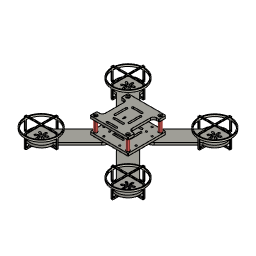
drone v11 (Autodesk Fusion 360 design; units mm, degrees)
Autodesk Fusion 360 part; units mm, degrees
(part 1 of 2)
sketch "Sketch1" plane through (0, 0, 0) normal (0, 0, 1) x (1, 0, 0)
  line L0 (0, 0) -> (74.2462, 0)
  line L1 (74.2462, 0) -> (74.2462, 74.2462)
  line L2 (74.2462, 74.2462) -> (0, 74.2462)
  line L3 (0, 74.2462) -> (0, 0)
  circle A0 centre (74.2462, 74.2462) radius 1
  circle A1 centre (0, 74.2462) radius 1
  circle A2 centre (0, 0) radius 1
  circle A3 centre (74.2462, 0) radius 1
  circle A4 centre (0, 74.2462) radius 10
  circle A5 centre (74.2462, 74.2462) radius 10
  circle A6 centre (74.2462, 0) radius 10
  circle A7 centre (0, 0) radius 10
  line L4 (59.6231, 14.6231) -> (14.6231, 14.6231)
  line L5 (14.6231, 14.6231) -> (14.6231, 59.6231)
  line L6 (14.6231, 59.6231) -> (59.6231, 59.6231)
  line L7 (59.6231, 59.6231) -> (59.6231, 14.6231)
  line L8 (59.6231, 14.6231) -> (14.6231, 59.6231) construction
  line L9 (14.6231, 14.6231) -> (59.6231, 59.6231) construction
  line L10 (0, 64.2462) -> (14.8037, 49.4426)
  line L11 (0, 64.2462) -> (20.9355, 64.2462) construction
  line L12 (10, 74.2462) -> (24.628, 59.6182)
  line L13 (10, 74.2462) -> (30.6871, 74.2462) construction
  line L14 (10, 0) -> (25.5198, 15.5198)
  line L15 (10, 0) -> (31.9483, 0) construction
  line L16 (0, 10) -> (14.6231, 24.6231)
  line L17 (0, 10) -> (20.6802, 10) construction
  line L18 (64.2462, 0) -> (49.6231, 14.6231)
  line L19 (74.2462, 10) -> (59.6231, 24.6231)
  line L20 (74.2462, 10) -> (94.9264, 10) construction
  line L21 (74.2462, 64.2462) -> (59.6231, 49.6231)
  line L22 (74.2462, 64.2462) -> (94.9264, 64.2462) construction
  line L23 (64.2462, 74.2462) -> (49.6231, 59.6231)
  line L24 (64.2462, 74.2462) -> (84.9264, 74.2462) construction
  point P0 (37.1231, 37.1231)
  dimension "d1" = 105
  dimension "d2" = 2
  dimension "d3" = 2
  dimension "d4" = 2
  dimension "d5" = 2
  dimension "d6" = 20
  dimension "d7" = 20
  dimension "d8" = 20
  dimension "d9" = 20
  dimension "d10" = 45
  dimension "d11" = 45
  dimension "d12" = 45
  constraint horizontal L0
  constraint vertical L1
  constraint horizontal L2
  constraint vertical L3
  constraint coincident L0.start L3.end
  constraint coincident L1.end L2.start
  constraint coincident L2.end L3.start
  constraint coincident L0.end L1.start
  constraint concentric A1 A4
  constraint concentric A0 A5
  constraint concentric A3 A6
  constraint concentric A2 A7
  constraint horizontal L4
  constraint perpendicular L4 L5
  constraint parallel L4 L6
  constraint parallel L5 L7
  constraint coincident L8 P0
  constraint coincident L9 P0
  constraint horizontal L11
  constraint coincident A4 L10.start
  constraint coincident L3 L10.start
  constraint horizontal L13
  constraint coincident A4 L12.start
  constraint coincident L2 L12.start
  constraint horizontal L15
  constraint coincident A7 L14.start
  constraint coincident L0 L14.start
  constraint horizontal L17
  constraint coincident A7 L16.start
  constraint coincident L3 L16.start
  constraint coincident L5 L16.end
  constraint coincident A6 L18.start
  constraint coincident L0 L18.start
  constraint coincident L4 L18.end
  constraint horizontal L20
  constraint coincident A6 L19.start
  constraint coincident L1 L19.start
  constraint coincident L7 L19.end
  constraint horizontal L22
  constraint coincident A5 L21.start
  constraint coincident L1 L21.start
  constraint coincident L7 L21.end
  constraint horizontal L24
  constraint coincident A5 L23.start
  constraint coincident L2 L23.start
  constraint coincident L6 L23.end
  measures "d1" distance of L0.start L1.end
  measures "d2" diameter of A0
  measures "d3" diameter of A1
  measures "d4" diameter of A2
  measures "d5" diameter of A3
  measures "d6" diameter of A4
  measures "d7" diameter of A5
  measures "d8" diameter of A6
  measures "d9" diameter of A7
  measures "d10" distance of L5.end L6.end
  measures "d11" distance of L4.end L5.end
  measures "d12" angle of L10 L11
extrude "Extrude1" add sketch "Sketch1" along normal blind 2 contours L0 L3 A2 A7 | L0 L3 A2 A7 | A7 L4 L5 L14 L16 | L0 L1 A3 A6 | A6 L4 L7 L18 L19 | L0 L1 A3 A6 | L4 L5 L6 L7 | L2 L3 A1 A4 | L2 L3 A1 A4 | A4 L5 L6 L10 L12 | L1 L2 A0 A5 | A5 L6 L7 L21 L23 | L1 L2 A0 A5 makes body 1
sketch "Sketch2" plane through (0, 0, 2) normal (0, 0, 1) x (-1, 0, 0)
  circle A0 centre (-74.2462, 0) radius 1
  circle A1 centre (0, -74.2462) radius 1
  circle A2 centre (0, 0) radius 1
  circle A3 centre (-74.2462, -74.2462) radius 1
  arc A4 (-74.2462, -64.2462) -> (-64.2462, -74.2462) centre (-74.2462, -74.2462) ccw
  line L0 (-64.2462, -74.2462) -> (-49.6231, -59.6231)
  line L1 (-49.6231, -59.6231) -> (-24.6231, -59.6231)
  line L2 (-24.6231, -59.6231) -> (-10, -74.2462)
  arc A5 (-10, -74.2462) -> (0, -64.2462) centre (0, -74.2462) ccw
  line L3 (0, -64.2462) -> (-14.6231, -49.6231)
  line L4 (-14.6231, -49.6231) -> (-14.6231, -24.6231)
  line L5 (-14.6231, -24.6231) -> (0, -10)
  arc A6 (0, -10) -> (-10, 0) centre (0, 0) ccw
  line L6 (-10, 0) -> (-24.6231, -14.6231)
  line L7 (-24.6231, -14.6231) -> (-49.6231, -14.6231)
  line L8 (-49.6231, -14.6231) -> (-64.2462, 0)
  arc A7 (-64.2462, 0) -> (-74.2462, -10) centre (-74.2462, 0) ccw
  line L9 (-74.2462, -10) -> (-59.6231, -24.6231)
  line L10 (-59.6231, -24.6231) -> (-59.6231, -49.6231)
  line L11 (-59.6231, -49.6231) -> (-74.2462, -64.2462)
  line L12 (0.7, -78.2462) -> (0.7, -76.5)
  arc A8 (0.7, -76.5) -> (-0.7, -76.5) centre (0, -76.5) ccw
  line L13 (-0.7, -76.5) -> (-0.7, -78.2462)
  arc A9 (-0.7, -78.2462) -> (0.7, -78.2462) centre (0, -78.2462) ccw
  line L14 (0, -78.2462) -> (0, -76.5) construction
  line L15 (3.8141, -75.64) -> (2.3018, -74.7669)
  arc A10 (3.1141, -76.8524) -> (3.8141, -75.64) centre (3.4641, -76.2462) ccw
  line L16 (1.6018, -75.9793) -> (3.1141, -76.8524)
  arc A11 (2.3018, -74.7669) -> (1.6018, -75.9793) centre (1.9518, -75.3731) ccw
  line L17 (3.1141, -71.64) -> (1.6018, -72.5131)
  arc A12 (3.8141, -72.8524) -> (3.1141, -71.64) centre (3.4641, -72.2462) ccw
  line L18 (2.3018, -73.7255) -> (3.8141, -72.8524)
  arc A13 (1.6018, -72.5131) -> (2.3018, -73.7255) centre (1.9518, -73.1193) ccw
  line L19 (-0.7, -70.2462) -> (-0.7, -71.9924)
  arc A14 (0.7, -70.2462) -> (-0.7, -70.2462) centre (0, -70.2462) ccw
  line L20 (0.7, -71.9924) -> (0.7, -70.2462)
  arc A15 (-0.7, -71.9924) -> (0.7, -71.9924) centre (0, -71.9924) ccw
  line L21 (-3.8141, -72.8524) -> (-2.3018, -73.7255)
  arc A16 (-3.1141, -71.64) -> (-3.8141, -72.8524) centre (-3.4641, -72.2462) ccw
  line L22 (-1.6018, -72.5131) -> (-3.1141, -71.64)
  arc A17 (-2.3018, -73.7255) -> (-1.6018, -72.5131) centre (-1.9518, -73.1193) ccw
  line L23 (-3.1141, -76.8524) -> (-1.6018, -75.9793)
  arc A18 (-3.8141, -75.64) -> (-3.1141, -76.8524) centre (-3.4641, -76.2462) ccw
  line L24 (-2.3018, -74.7669) -> (-3.8141, -75.64)
  arc A19 (-1.6018, -75.9793) -> (-2.3018, -74.7669) centre (-1.9518, -75.3731) ccw
  line L25 (-74.9462, -78.2462) -> (-74.9462, -76.5)
  line L26 (-74.9462, -71.9924) -> (-74.9462, -70.2462)
  arc A20 (-78.0603, -75.64) -> (-77.3603, -76.8524) centre (-77.7103, -76.2462) ccw
  arc A21 (-73.5462, -76.5) -> (-74.9462, -76.5) centre (-74.2462, -76.5) ccw
  line L27 (-78.0603, -75.64) -> (-76.5481, -74.7669)
  line L28 (-72.6444, -72.5131) -> (-71.1321, -71.64)
  line L29 (-73.5462, -76.5) -> (-73.5462, -78.2462)
  arc A22 (-77.3603, -71.64) -> (-78.0603, -72.8524) centre (-77.7103, -72.2462) ccw
  arc A23 (-74.9462, -78.2462) -> (-73.5462, -78.2462) centre (-74.2462, -78.2462) ccw
  arc A24 (-72.6444, -72.5131) -> (-71.9444, -73.7255) centre (-72.2944, -73.1193) ccw
  arc A25 (-71.1321, -76.8524) -> (-70.4321, -75.64) centre (-70.7821, -76.2462) ccw
  line L30 (-77.3603, -71.64) -> (-75.8481, -72.5131)
  arc A26 (-71.9444, -74.7669) -> (-72.6444, -75.9793) centre (-72.2944, -75.3731) ccw
  arc A27 (-74.9462, -71.9924) -> (-73.5462, -71.9924) centre (-74.2462, -71.9924) ccw
  line L31 (-73.5462, -70.2462) -> (-73.5462, -71.9924)
  line L32 (-71.1321, -76.8524) -> (-72.6444, -75.9793)
  arc A28 (-76.5481, -73.7255) -> (-75.8481, -72.5131) centre (-76.1981, -73.1193) ccw
  line L33 (-75.8481, -75.9793) -> (-77.3603, -76.8524)
  line L34 (-74.2462, -78.2462) -> (-74.2462, -76.5) construction
  line L35 (-70.4321, -72.8524) -> (-71.9444, -73.7255)
  line L36 (-71.9444, -74.7669) -> (-70.4321, -75.64)
  circle A29 centre (-74.2462, -74.2462) radius 1
  arc A30 (-73.5462, -70.2462) -> (-74.9462, -70.2462) centre (-74.2462, -70.2462) ccw
  arc A31 (-70.4321, -72.8524) -> (-71.1321, -71.64) centre (-70.7821, -72.2462) ccw
  line L37 (-76.5481, -73.7255) -> (-78.0603, -72.8524)
  arc A32 (-75.8481, -75.9793) -> (-76.5481, -74.7669) centre (-76.1981, -75.3731) ccw
  arc A33 (-0.7, -4) -> (0.7, -4) centre (0, -4) ccw
  arc A34 (0.7, 4) -> (-0.7, 4) centre (0, 4) ccw
  arc A35 (1.6018, 1.7331) -> (2.3018, 0.5207) centre (1.9518, 1.1269) ccw
  line L38 (1.6018, 1.7331) -> (3.1141, 2.6062)
  line L39 (-3.8141, -1.3938) -> (-2.3018, -0.5207)
  line L40 (-1.6018, -1.7331) -> (-3.1141, -2.6062)
  arc A36 (2.3018, -0.5207) -> (1.6018, -1.7331) centre (1.9518, -1.1269) ccw
  line L41 (3.1141, -2.6062) -> (1.6018, -1.7331)
  arc A37 (-0.7, 2.2538) -> (0.7, 2.2538) centre (0, 2.2538) ccw
  line L42 (2.3018, -0.5207) -> (3.8141, -1.3938)
  arc A38 (-3.1141, 2.6062) -> (-3.8141, 1.3938) centre (-3.4641, 2) ccw
  line L43 (3.8141, 1.3938) -> (2.3018, 0.5207)
  arc A39 (0.7, -2.2538) -> (-0.7, -2.2538) centre (0, -2.2538) ccw
  line L44 (0.7, 4) -> (0.7, 2.2538)
  arc A40 (3.1141, -2.6062) -> (3.8141, -1.3938) centre (3.4641, -2) ccw
  arc A41 (-3.8141, -1.3938) -> (-3.1141, -2.6062) centre (-3.4641, -2) ccw
  line L45 (-0.7, -4) -> (-0.7, -2.2538)
  line L46 (-3.1141, 2.6062) -> (-1.6018, 1.7331)
  circle A42 centre (0, 0) radius 1
  line L47 (0, 4) -> (0, 2.2538) construction
  arc A43 (3.8141, 1.3938) -> (3.1141, 2.6062) centre (3.4641, 2) ccw
  line L48 (-0.7, 2.2538) -> (-0.7, 4)
  line L49 (-2.3018, 0.5207) -> (-3.8141, 1.3938)
  arc A44 (-2.3018, 0.5207) -> (-1.6018, 1.7331) centre (-1.9518, 1.1269) ccw
  arc A45 (-1.6018, -1.7331) -> (-2.3018, -0.5207) centre (-1.9518, -1.1269) ccw
  line L50 (0.7, -2.2538) -> (0.7, -4)
  line L51 (-75.8481, 1.7331) -> (-77.3603, 2.6062)
  line L52 (-73.5462, 2.2538) -> (-73.5462, 4)
  arc A46 (-72.6444, 1.7331) -> (-71.9444, 0.5207) centre (-72.2944, 1.1269) ccw
  line L53 (-78.0603, 1.3938) -> (-76.5481, 0.5207)
  line L54 (-77.3603, -2.6062) -> (-75.8481, -1.7331)
  arc A47 (-71.9444, -0.5207) -> (-72.6444, -1.7331) centre (-72.2944, -1.1269) ccw
  arc A48 (-74.9462, -4) -> (-73.5462, -4) centre (-74.2462, -4) ccw
  line L55 (-71.9444, 0.5207) -> (-70.4321, 1.3938)
  arc A49 (-77.3603, 2.6062) -> (-78.0603, 1.3938) centre (-77.7103, 2) ccw
  line L56 (-72.6444, -1.7331) -> (-71.1321, -2.6062)
  circle A50 centre (-74.2462, 0) radius 1
  line L57 (-70.4321, -1.3938) -> (-71.9444, -0.5207)
  arc A51 (-71.1321, -2.6062) -> (-70.4321, -1.3938) centre (-70.7821, -2) ccw
  arc A52 (-78.0603, -1.3938) -> (-77.3603, -2.6062) centre (-77.7103, -2) ccw
  arc A53 (-75.8481, -1.7331) -> (-76.5481, -0.5207) centre (-76.1981, -1.1269) ccw
  arc A54 (-73.5462, -2.2538) -> (-74.9462, -2.2538) centre (-74.2462, -2.2538) ccw
  line L58 (-74.9462, 4) -> (-74.9462, 2.2538)
  circle A55 centre (-74.2462, 0) radius 1
  line L59 (-76.5481, -0.5207) -> (-78.0603, -1.3938)
  line L60 (-71.1321, 2.6062) -> (-72.6444, 1.7331)
  line L61 (-73.5462, -4) -> (-73.5462, -2.2538)
  arc A56 (-70.4321, 1.3938) -> (-71.1321, 2.6062) centre (-70.7821, 2) ccw
  line L62 (-74.9462, -2.2538) -> (-74.9462, -4)
  arc A57 (-74.9462, 2.2538) -> (-73.5462, 2.2538) centre (-74.2462, 2.2538) ccw
  arc A58 (-76.5481, 0.5207) -> (-75.8481, 1.7331) centre (-76.1981, 1.1269) ccw
  arc A59 (-73.5462, 4) -> (-74.9462, 4) centre (-74.2462, 4) ccw
  line L63 (-74.2462, 4) -> (-74.2462, 2.2538) construction
  dimension "d32" = 1.4
  constraint tangent L12 A8
  constraint tangent A8 L13
  constraint parallel L12 L13
  constraint tangent L13 A9
  constraint tangent L12 A9
  measures "d32" diameter of A8
extrude "Extrude2" cut sketch "Sketch2" against normal blind 5 contours L12 A8 L13 A9 | L15 A10 L16 A11 | L17 A12 L18 A13 | L19 A14 L20 A15 | L21 A16 L22 A17 | L23 A18 L24 A19 | L25 A21 L29 A23 | L26 A27 L31 A30 | A20 L27 L33 A32 | L28 A24 L35 A31 | A22 L30 A28 L37 | A25 A26 L32 L36 | A33 A39 L45 L50 | A34 A37 L44 L48 | A35 L38 L43 A43 | L39 L40 A41 A45 | A36 L41 L42 A40 | A38 L46 L49 A44 | L51 L53 A49 A58 | L52 L58 A57 A59 | A46 L55 L60 A56 | L54 A52 A53 L59 | A47 L56 L57 A51 | A48 A54 L61 L62 bodies 1
sketch "Sketch3" plane through (0, 0, 2) normal (0, 0, 1) x (-1, 0, 0)
  line L0 (-0.7, 2.2538) -> (-0.7, 4)
  arc A0 (0.7, 4) -> (-0.7, 4) centre (0, 4) ccw
  line L1 (0.7, 4) -> (0.7, 2.2538)
  arc A1 (-0.7, 2.2538) -> (0.7, 2.2538) centre (0, 2.2538) ccw
  line L2 (-72.6444, 1.7331) -> (-71.1321, 2.6062)
  arc A2 (-70.4321, 1.3938) -> (-71.1321, 2.6062) centre (-70.7821, 2) ccw
  line L3 (-70.4321, 1.3938) -> (-71.9444, 0.5207)
  arc A3 (-72.6444, 1.7331) -> (-71.9444, 0.5207) centre (-72.2944, 1.1269) ccw
  arc A4 (-74.9462, -4) -> (-73.5462, -4) centre (-74.2462, -4) ccw
  line L4 (-74.9462, -4) -> (-74.9462, -2.2538)
  arc A5 (-73.5462, -2.2538) -> (-74.9462, -2.2538) centre (-74.2462, -2.2538) ccw
  line L5 (-73.5462, -2.2538) -> (-73.5462, -4)
  line L6 (-76.5481, -73.7255) -> (-78.0603, -72.8524)
  arc A6 (-77.3603, -71.64) -> (-78.0603, -72.8524) centre (-77.7103, -72.2462) ccw
  line L7 (-77.3603, -71.64) -> (-75.8481, -72.5131)
  arc A7 (-76.5481, -73.7255) -> (-75.8481, -72.5131) centre (-76.1981, -73.1193) ccw
  line L8 (3.8141, -72.8524) -> (2.3018, -73.7255)
  arc A8 (1.6018, -72.5131) -> (2.3018, -73.7255) centre (1.9518, -73.1193) ccw
  line L9 (1.6018, -72.5131) -> (3.1141, -71.64)
  arc A9 (3.8141, -72.8524) -> (3.1141, -71.64) centre (3.4641, -72.2462) ccw
  line L10 (0.7, -76.5) -> (0.7, -78.2462)
  arc A10 (-0.7, -78.2462) -> (0.7, -78.2462) centre (0, -78.2462) ccw
  line L11 (-0.7, -78.2462) -> (-0.7, -76.5)
  arc A11 (0.7, -76.5) -> (-0.7, -76.5) centre (0, -76.5) ccw
  line L12 (-3.8141, -75.64) -> (-2.3018, -74.7669)
  arc A12 (-1.6018, -75.9793) -> (-2.3018, -74.7669) centre (-1.9518, -75.3731) ccw
  line L13 (-1.6018, -75.9793) -> (-3.1141, -76.8524)
  arc A13 (-3.8141, -75.64) -> (-3.1141, -76.8524) centre (-3.4641, -76.2462) ccw
  line L14 (-71.9444, -74.7669) -> (-70.4321, -75.64)
  arc A14 (-71.1321, -76.8524) -> (-70.4321, -75.64) centre (-70.7821, -76.2462) ccw
  line L15 (-71.1321, -76.8524) -> (-72.6444, -75.9793)
  arc A15 (-71.9444, -74.7669) -> (-72.6444, -75.9793) centre (-72.2944, -75.3731) ccw
  line L16 (-70.4321, -72.8524) -> (-71.9444, -73.7255)
  arc A16 (-72.6444, -72.5131) -> (-71.9444, -73.7255) centre (-72.2944, -73.1193) ccw
  line L17 (-72.6444, -72.5131) -> (-71.1321, -71.64)
  arc A17 (-70.4321, -72.8524) -> (-71.1321, -71.64) centre (-70.7821, -72.2462) ccw
  arc A18 (-78.0603, -1.3938) -> (-77.3603, -2.6062) centre (-77.7103, -2) ccw
  line L18 (-78.0603, -1.3938) -> (-76.5481, -0.5207)
  arc A19 (-75.8481, -1.7331) -> (-76.5481, -0.5207) centre (-76.1981, -1.1269) ccw
  line L19 (-75.8481, -1.7331) -> (-77.3603, -2.6062)
  line L20 (0.7, -2.2538) -> (0.7, -4)
  arc A20 (-0.7, -4) -> (0.7, -4) centre (0, -4) ccw
  line L21 (-0.7, -4) -> (-0.7, -2.2538)
  arc A21 (0.7, -2.2538) -> (-0.7, -2.2538) centre (0, -2.2538) ccw
  line L22 (3.8141, 1.3938) -> (2.3018, 0.5207)
  arc A22 (1.6018, 1.7331) -> (2.3018, 0.5207) centre (1.9518, 1.1269) ccw
  line L23 (1.6018, 1.7331) -> (3.1141, 2.6062)
  arc A23 (3.8141, 1.3938) -> (3.1141, 2.6062) centre (3.4641, 2) ccw
  line L24 (-2.3018, 0.5207) -> (-3.8141, 1.3938)
  arc A24 (-3.1141, 2.6062) -> (-3.8141, 1.3938) centre (-3.4641, 2) ccw
  line L25 (-3.1141, 2.6062) -> (-1.6018, 1.7331)
  arc A25 (-2.3018, 0.5207) -> (-1.6018, 1.7331) centre (-1.9518, 1.1269) ccw
  line L26 (-74.9462, 2.2538) -> (-74.9462, 4)
  arc A26 (-73.5462, 4) -> (-74.9462, 4) centre (-74.2462, 4) ccw
  line L27 (-73.5462, 4) -> (-73.5462, 2.2538)
  arc A27 (-74.9462, 2.2538) -> (-73.5462, 2.2538) centre (-74.2462, 2.2538) ccw
  line L28 (-71.9444, -0.5207) -> (-70.4321, -1.3938)
  arc A28 (-71.1321, -2.6062) -> (-70.4321, -1.3938) centre (-70.7821, -2) ccw
  line L29 (-71.1321, -2.6062) -> (-72.6444, -1.7331)
  arc A29 (-71.9444, -0.5207) -> (-72.6444, -1.7331) centre (-72.2944, -1.1269) ccw
  line L30 (-75.8481, -75.9793) -> (-77.3603, -76.8524)
  arc A30 (-78.0603, -75.64) -> (-77.3603, -76.8524) centre (-77.7103, -76.2462) ccw
  line L31 (-78.0603, -75.64) -> (-76.5481, -74.7669)
  arc A31 (-75.8481, -75.9793) -> (-76.5481, -74.7669) centre (-76.1981, -75.3731) ccw
  line L32 (0.7, -70.2462) -> (0.7, -71.9924)
  arc A32 (-0.7, -71.9924) -> (0.7, -71.9924) centre (0, -71.9924) ccw
  line L33 (-0.7, -71.9924) -> (-0.7, -70.2462)
  arc A33 (0.7, -70.2462) -> (-0.7, -70.2462) centre (0, -70.2462) ccw
  line L34 (3.1141, -76.8524) -> (1.6018, -75.9793)
  arc A34 (2.3018, -74.7669) -> (1.6018, -75.9793) centre (1.9518, -75.3731) ccw
  line L35 (2.3018, -74.7669) -> (3.8141, -75.64)
  arc A35 (3.1141, -76.8524) -> (3.8141, -75.64) centre (3.4641, -76.2462) ccw
  line L36 (-3.1141, -71.64) -> (-1.6018, -72.5131)
  arc A36 (-2.3018, -73.7255) -> (-1.6018, -72.5131) centre (-1.9518, -73.1193) ccw
  line L37 (-2.3018, -73.7255) -> (-3.8141, -72.8524)
  arc A37 (-3.1141, -71.64) -> (-3.8141, -72.8524) centre (-3.4641, -72.2462) ccw
  line L38 (-74.9462, -78.2462) -> (-74.9462, -76.5)
  arc A38 (-73.5462, -76.5) -> (-74.9462, -76.5) centre (-74.2462, -76.5) ccw
  line L39 (-73.5462, -76.5) -> (-73.5462, -78.2462)
  arc A39 (-74.9462, -78.2462) -> (-73.5462, -78.2462) centre (-74.2462, -78.2462) ccw
  line L40 (-73.5462, -70.2462) -> (-73.5462, -71.9924)
  arc A40 (-74.9462, -71.9924) -> (-73.5462, -71.9924) centre (-74.2462, -71.9924) ccw
  line L41 (-74.9462, -71.9924) -> (-74.9462, -70.2462)
  arc A41 (-73.5462, -70.2462) -> (-74.9462, -70.2462) centre (-74.2462, -70.2462) ccw
  line L42 (-77.3603, 2.6062) -> (-75.8481, 1.7331)
  arc A42 (-76.5481, 0.5207) -> (-75.8481, 1.7331) centre (-76.1981, 1.1269) ccw
  line L43 (-76.5481, 0.5207) -> (-78.0603, 1.3938)
  arc A43 (-77.3603, 2.6062) -> (-78.0603, 1.3938) centre (-77.7103, 2) ccw
  line L44 (-1.6018, -1.7331) -> (-3.1141, -2.6062)
  arc A44 (-3.8141, -1.3938) -> (-3.1141, -2.6062) centre (-3.4641, -2) ccw
  line L45 (-3.8141, -1.3938) -> (-2.3018, -0.5207)
  arc A45 (-1.6018, -1.7331) -> (-2.3018, -0.5207) centre (-1.9518, -1.1269) ccw
  line L46 (3.1141, -2.6062) -> (1.6018, -1.7331)
  arc A46 (2.3018, -0.5207) -> (1.6018, -1.7331) centre (1.9518, -1.1269) ccw
  line L47 (2.3018, -0.5207) -> (3.8141, -1.3938)
  arc A47 (3.1141, -2.6062) -> (3.8141, -1.3938) centre (3.4641, -2) ccw
  circle A48 centre (-74.2462, 0) radius 1
  circle A49 centre (0, -74.2462) radius 1
  circle A50 centre (0, 0) radius 1
  circle A51 centre (-74.2462, -74.2462) radius 1
  arc A52 (-74.2462, -64.2462) -> (-64.2462, -74.2462) centre (-74.2462, -74.2462) ccw
  line L48 (-64.2462, -74.2462) -> (-49.6231, -59.6231)
  line L49 (-49.6231, -59.6231) -> (-24.6231, -59.6231)
  line L50 (-24.6231, -59.6231) -> (-10, -74.2462)
  arc A53 (-10, -74.2462) -> (0, -64.2462) centre (0, -74.2462) ccw
  line L51 (0, -64.2462) -> (-14.6231, -49.6231)
  line L52 (-14.6231, -49.6231) -> (-14.6231, -24.6231)
  line L53 (-14.6231, -24.6231) -> (0, -10)
  arc A54 (0, -10) -> (-10, 0) centre (0, 0) ccw
  line L54 (-10, 0) -> (-24.6231, -14.6231)
  line L55 (-24.6231, -14.6231) -> (-49.6231, -14.6231)
  line L56 (-49.6231, -14.6231) -> (-64.2462, 0)
  arc A55 (-64.2462, 0) -> (-74.2462, -10) centre (-74.2462, 0) ccw
  line L57 (-74.2462, -10) -> (-59.6231, -24.6231)
  line L58 (-59.6231, -24.6231) -> (-59.6231, -49.6231)
  line L59 (-59.6231, -49.6231) -> (-74.2462, -64.2462)
  line L60 (-49.6231, -59.6231) -> (-14.6231, -24.6231)
  line L61 (-49.6231, -59.6231) -> (-0.1256, -59.6231) construction
  line L62 (-24.6231, -59.6231) -> (-59.6231, -24.6231)
  line L63 (-24.6231, -14.6231) -> (-59.6231, -49.6231)
  line L64 (-49.6231, -14.6231) -> (-14.6231, -49.6231)
  line L65 (-20.8731, -37.1231) -> (-20.8731, -30.8731)
  line L66 (-20.8731, -30.8731) -> (-20.8731, -43.3731)
  line L67 (-37.1231, -20.8731) -> (-43.3731, -20.8731)
  line L68 (-43.3731, -20.8731) -> (-30.8731, -20.8731)
  line L69 (-53.3731, -37.1231) -> (-53.3731, -30.8731)
  line L70 (-53.3731, -30.8731) -> (-53.3731, -43.3731)
  line L71 (-37.1231, -53.3731) -> (-43.3731, -53.3731)
  line L72 (-43.3731, -53.3731) -> (-30.8731, -53.3731)
  dimension "d37" = 45
  constraint horizontal L61
  constraint coincident L48.end L49.start
  constraint coincident L52 L53.start
  constraint coincident L49.end L50.start
  constraint coincident L57.end L58.start
  constraint coincident L54.end L55.start
  constraint coincident L58.end L59.start
  constraint coincident L55.end L56.start
  constraint coincident L51.end L52.start
  constraint coincident L60 L65.end
  constraint coincident L64 L66.end
  constraint coincident L64 L67.end
  constraint coincident L63 L68.end
  constraint coincident L62 L69.end
  constraint coincident L63 L70.end
  constraint coincident L60 L71.end
  constraint coincident L62 L72.end
  measures "d37" angle of L60 L61
extrude "Extrude3" cut sketch "Sketch3" against normal blind 10 contours L58 L62 L63 L69 L70 | L49 L60 L62 L71 L72 | L55 L63 L64 L67 L68 | L52 L60 L64 L65 L66 bodies 1
sketch "Sketch4" plane through (0, 0, 2) normal (0, 0, 1) x (-1, 0, 0)
  line L0 (-30.8731, -53.3731) -> (-10, -74.2462)
  arc A0 (-10, -74.2462) -> (0, -64.2462) centre (0, -74.2462) ccw
  line L1 (0, -64.2462) -> (-20.8731, -43.3731)
  line L2 (-20.8731, -43.3731) -> (-20.8731, -30.8731)
  line L3 (-20.8731, -30.8731) -> (0, -10)
  arc A1 (0, -10) -> (-10, 0) centre (0, 0) ccw
  line L4 (-10, 0) -> (-30.8731, -20.8731)
  line L5 (-30.8731, -20.8731) -> (-43.3731, -20.8731)
  line L6 (-43.3731, -20.8731) -> (-64.2462, 0)
  arc A2 (-64.2462, 0) -> (-74.2462, -10) centre (-74.2462, 0) ccw
  line L7 (-74.2462, -10) -> (-53.3731, -30.8731)
  line L8 (-53.3731, -30.8731) -> (-53.3731, -43.3731)
  line L9 (-53.3731, -43.3731) -> (-74.2462, -64.2462)
  arc A3 (-74.2462, -64.2462) -> (-64.2462, -74.2462) centre (-74.2462, -74.2462) ccw
  line L10 (-64.2462, -74.2462) -> (-43.3731, -53.3731)
  line L11 (-43.3731, -53.3731) -> (-30.8731, -53.3731)
  line L12 (-0.7, 2.2538) -> (-0.7, 4)
  arc A4 (0.7, 4) -> (-0.7, 4) centre (0, 4) ccw
  line L13 (0.7, 4) -> (0.7, 2.2538)
  arc A5 (-0.7, 2.2538) -> (0.7, 2.2538) centre (0, 2.2538) ccw
  line L14 (-72.6444, 1.7331) -> (-71.1321, 2.6062)
  arc A6 (-70.4321, 1.3938) -> (-71.1321, 2.6062) centre (-70.7821, 2) ccw
  line L15 (-70.4321, 1.3938) -> (-71.9444, 0.5207)
  arc A7 (-72.6444, 1.7331) -> (-71.9444, 0.5207) centre (-72.2944, 1.1269) ccw
  arc A8 (-74.9462, -4) -> (-73.5462, -4) centre (-74.2462, -4) ccw
  line L16 (-74.9462, -4) -> (-74.9462, -2.2538)
  arc A9 (-73.5462, -2.2538) -> (-74.9462, -2.2538) centre (-74.2462, -2.2538) ccw
  line L17 (-73.5462, -2.2538) -> (-73.5462, -4)
  line L18 (-76.5481, -73.7255) -> (-78.0603, -72.8524)
  arc A10 (-77.3603, -71.64) -> (-78.0603, -72.8524) centre (-77.7103, -72.2462) ccw
  line L19 (-77.3603, -71.64) -> (-75.8481, -72.5131)
  arc A11 (-76.5481, -73.7255) -> (-75.8481, -72.5131) centre (-76.1981, -73.1193) ccw
  line L20 (3.8141, -72.8524) -> (2.3018, -73.7255)
  arc A12 (1.6018, -72.5131) -> (2.3018, -73.7255) centre (1.9518, -73.1193) ccw
  line L21 (1.6018, -72.5131) -> (3.1141, -71.64)
  arc A13 (3.8141, -72.8524) -> (3.1141, -71.64) centre (3.4641, -72.2462) ccw
  line L22 (0.7, -76.5) -> (0.7, -78.2462)
  arc A14 (-0.7, -78.2462) -> (0.7, -78.2462) centre (0, -78.2462) ccw
  line L23 (-0.7, -78.2462) -> (-0.7, -76.5)
  arc A15 (0.7, -76.5) -> (-0.7, -76.5) centre (0, -76.5) ccw
  line L24 (-3.8141, -75.64) -> (-2.3018, -74.7669)
  arc A16 (-1.6018, -75.9793) -> (-2.3018, -74.7669) centre (-1.9518, -75.3731) ccw
  line L25 (-1.6018, -75.9793) -> (-3.1141, -76.8524)
  arc A17 (-3.8141, -75.64) -> (-3.1141, -76.8524) centre (-3.4641, -76.2462) ccw
  line L26 (-71.9444, -74.7669) -> (-70.4321, -75.64)
  arc A18 (-71.1321, -76.8524) -> (-70.4321, -75.64) centre (-70.7821, -76.2462) ccw
  line L27 (-71.1321, -76.8524) -> (-72.6444, -75.9793)
  arc A19 (-71.9444, -74.7669) -> (-72.6444, -75.9793) centre (-72.2944, -75.3731) ccw
  line L28 (-70.4321, -72.8524) -> (-71.9444, -73.7255)
  arc A20 (-72.6444, -72.5131) -> (-71.9444, -73.7255) centre (-72.2944, -73.1193) ccw
  line L29 (-72.6444, -72.5131) -> (-71.1321, -71.64)
  arc A21 (-70.4321, -72.8524) -> (-71.1321, -71.64) centre (-70.7821, -72.2462) ccw
  arc A22 (-78.0603, -1.3938) -> (-77.3603, -2.6062) centre (-77.7103, -2) ccw
  line L30 (-78.0603, -1.3938) -> (-76.5481, -0.5207)
  arc A23 (-75.8481, -1.7331) -> (-76.5481, -0.5207) centre (-76.1981, -1.1269) ccw
  line L31 (-75.8481, -1.7331) -> (-77.3603, -2.6062)
  line L32 (0.7, -2.2538) -> (0.7, -4)
  arc A24 (-0.7, -4) -> (0.7, -4) centre (0, -4) ccw
  line L33 (-0.7, -4) -> (-0.7, -2.2538)
  arc A25 (0.7, -2.2538) -> (-0.7, -2.2538) centre (0, -2.2538) ccw
  line L34 (3.8141, 1.3938) -> (2.3018, 0.5207)
  arc A26 (1.6018, 1.7331) -> (2.3018, 0.5207) centre (1.9518, 1.1269) ccw
  line L35 (1.6018, 1.7331) -> (3.1141, 2.6062)
  arc A27 (3.8141, 1.3938) -> (3.1141, 2.6062) centre (3.4641, 2) ccw
  line L36 (-2.3018, 0.5207) -> (-3.8141, 1.3938)
  arc A28 (-3.1141, 2.6062) -> (-3.8141, 1.3938) centre (-3.4641, 2) ccw
  line L37 (-3.1141, 2.6062) -> (-1.6018, 1.7331)
  arc A29 (-2.3018, 0.5207) -> (-1.6018, 1.7331) centre (-1.9518, 1.1269) ccw
  line L38 (-74.9462, 2.2538) -> (-74.9462, 4)
  arc A30 (-73.5462, 4) -> (-74.9462, 4) centre (-74.2462, 4) ccw
  line L39 (-73.5462, 4) -> (-73.5462, 2.2538)
  arc A31 (-74.9462, 2.2538) -> (-73.5462, 2.2538) centre (-74.2462, 2.2538) ccw
  line L40 (-71.9444, -0.5207) -> (-70.4321, -1.3938)
  arc A32 (-71.1321, -2.6062) -> (-70.4321, -1.3938) centre (-70.7821, -2) ccw
  line L41 (-71.1321, -2.6062) -> (-72.6444, -1.7331)
  arc A33 (-71.9444, -0.5207) -> (-72.6444, -1.7331) centre (-72.2944, -1.1269) ccw
  line L42 (-75.8481, -75.9793) -> (-77.3603, -76.8524)
  arc A34 (-78.0603, -75.64) -> (-77.3603, -76.8524) centre (-77.7103, -76.2462) ccw
  line L43 (-78.0603, -75.64) -> (-76.5481, -74.7669)
  arc A35 (-75.8481, -75.9793) -> (-76.5481, -74.7669) centre (-76.1981, -75.3731) ccw
  line L44 (0.7, -70.2462) -> (0.7, -71.9924)
  arc A36 (-0.7, -71.9924) -> (0.7, -71.9924) centre (0, -71.9924) ccw
  line L45 (-0.7, -71.9924) -> (-0.7, -70.2462)
  arc A37 (0.7, -70.2462) -> (-0.7, -70.2462) centre (0, -70.2462) ccw
  line L46 (3.1141, -76.8524) -> (1.6018, -75.9793)
  arc A38 (2.3018, -74.7669) -> (1.6018, -75.9793) centre (1.9518, -75.3731) ccw
  line L47 (2.3018, -74.7669) -> (3.8141, -75.64)
  arc A39 (3.1141, -76.8524) -> (3.8141, -75.64) centre (3.4641, -76.2462) ccw
  line L48 (-3.1141, -71.64) -> (-1.6018, -72.5131)
  arc A40 (-2.3018, -73.7255) -> (-1.6018, -72.5131) centre (-1.9518, -73.1193) ccw
  line L49 (-2.3018, -73.7255) -> (-3.8141, -72.8524)
  arc A41 (-3.1141, -71.64) -> (-3.8141, -72.8524) centre (-3.4641, -72.2462) ccw
  line L50 (-74.9462, -78.2462) -> (-74.9462, -76.5)
  arc A42 (-73.5462, -76.5) -> (-74.9462, -76.5) centre (-74.2462, -76.5) ccw
  line L51 (-73.5462, -76.5) -> (-73.5462, -78.2462)
  arc A43 (-74.9462, -78.2462) -> (-73.5462, -78.2462) centre (-74.2462, -78.2462) ccw
  line L52 (-73.5462, -70.2462) -> (-73.5462, -71.9924)
  arc A44 (-74.9462, -71.9924) -> (-73.5462, -71.9924) centre (-74.2462, -71.9924) ccw
  line L53 (-74.9462, -71.9924) -> (-74.9462, -70.2462)
  arc A45 (-73.5462, -70.2462) -> (-74.9462, -70.2462) centre (-74.2462, -70.2462) ccw
  line L54 (-77.3603, 2.6062) -> (-75.8481, 1.7331)
  arc A46 (-76.5481, 0.5207) -> (-75.8481, 1.7331) centre (-76.1981, 1.1269) ccw
  line L55 (-76.5481, 0.5207) -> (-78.0603, 1.3938)
  arc A47 (-77.3603, 2.6062) -> (-78.0603, 1.3938) centre (-77.7103, 2) ccw
  line L56 (-1.6018, -1.7331) -> (-3.1141, -2.6062)
  arc A48 (-3.8141, -1.3938) -> (-3.1141, -2.6062) centre (-3.4641, -2) ccw
  line L57 (-3.8141, -1.3938) -> (-2.3018, -0.5207)
  arc A49 (-1.6018, -1.7331) -> (-2.3018, -0.5207) centre (-1.9518, -1.1269) ccw
  line L58 (3.1141, -2.6062) -> (1.6018, -1.7331)
  arc A50 (2.3018, -0.5207) -> (1.6018, -1.7331) centre (1.9518, -1.1269) ccw
  line L59 (2.3018, -0.5207) -> (3.8141, -1.3938)
  arc A51 (3.1141, -2.6062) -> (3.8141, -1.3938) centre (3.4641, -2) ccw
  circle A52 centre (-74.2462, 0) radius 1
  circle A53 centre (0, -74.2462) radius 1
  circle A54 centre (0, 0) radius 1
  circle A55 centre (-74.2462, -74.2462) radius 1
  line L60 (-30.8731, -53.3731) -> (-20.8731, -43.3731)
  arc A56 (-20.8731, -43.3731) -> (-30.8731, -53.3731) centre (-25.8731, -48.3731) ccw
  line L61 (-37.1231, -53.3731) -> (-37.1231, -20.8731)
  line L62 (-20.8731, -37.1231) -> (-53.3731, -37.1231)
  arc A57 (-43.3731, -53.3731) -> (-53.3731, -43.3731) centre (-48.3731, -48.3731) ccw
  line L63 (-43.3731, -53.3731) -> (-53.3731, -43.3731)
  arc A58 (-30.8731, -20.8731) -> (-20.8731, -30.8731) centre (-25.8731, -25.8731) ccw
  line L64 (-30.8731, -20.8731) -> (-20.8731, -30.8731)
  arc A59 (-53.3731, -30.8731) -> (-43.3731, -20.8731) centre (-48.3731, -25.8731) ccw
  line L65 (-43.3731, -20.8731) -> (-53.3731, -30.8731)
  line L66 (-43.3731, -53.3731) -> (-53.3731, -53.3731)
  line L67 (-53.3731, -53.3731) -> (-53.3731, -43.3731)
  line L68 (-30.8731, -53.3731) -> (-20.8731, -53.3731)
  line L69 (-20.8731, -53.3731) -> (-20.8731, -43.3731)
  line L70 (-30.8731, -20.8731) -> (-20.8731, -20.8731)
  line L71 (-20.8731, -20.8731) -> (-20.8731, -30.8731)
  line L72 (-43.3731, -20.8731) -> (-53.3731, -20.8731)
  line L73 (-53.3731, -20.8731) -> (-53.3731, -30.8731)
  circle A60 centre (-51, -51) radius 0.75
  circle A61 centre (-45, -45) radius 0.75
  circle A62 centre (-44, -51) radius 0.75
  circle A63 centre (-51, -44) radius 0.75
  circle A64 centre (-29.2462, -45) radius 0.75
  circle A65 centre (-30.2462, -51) radius 0.75
  circle A66 centre (-23.2462, -51) radius 0.75
  circle A67 centre (-23.2462, -44) radius 0.75
  circle A68 centre (-29.2462, -29.2462) radius 0.75
  circle A69 centre (-30.2462, -23.2462) radius 0.75
  circle A70 centre (-44, -23.2462) radius 0.75
  circle A71 centre (-51, -23.2462) radius 0.75
  circle A72 centre (-51, -30.2462) radius 0.75
  circle A73 centre (-45, -29.2462) radius 0.75
  circle A74 centre (-23.2462, -23.2462) radius 0.75
  circle A75 centre (-23.2462, -30.2462) radius 0.75
  dimension "d47" = 1.5
  dimension "d48" = 1.5
  dimension "d49" = 1.5
  dimension "d50" = 1.5
  constraint coincident L0.start L11.end
  constraint coincident L1.end L2.start
  constraint tangent L0 A56
  constraint midpoint L11 L61.start
  constraint midpoint L5 L61.end
  constraint midpoint L2 L62.start
  constraint midpoint L8 L62.end
  constraint symmetric L0.start L61 L10.end
  constraint symmetric L1.end L61 L8.end
  constraint symmetric A56 L61 A57
  constraint symmetric L0.start L62 L4.end
  constraint symmetric L1.end L62 L2.end
  constraint symmetric A56 L62 A58
  constraint symmetric L62 L8.end L7.end
  constraint symmetric L62 L10.end L5.end
  constraint symmetric L62 A57 A59
  constraint coincident L10.end L11.start
  constraint horizontal L66
  constraint perpendicular L66 L67
  constraint symmetric L61 L8.end L1.end
  constraint symmetric L61 L10.end L0.start
  constraint symmetric L61 L66.end L68.end
  constraint symmetric L62 L66.end L72.end
  constraint symmetric L62 L0.start L4.end
  constraint symmetric L62 L68.end L70.end
  constraint symmetric L62 L1.end L2.end
  constraint symmetric L61 A60 A66
  constraint symmetric L61 A61 A64
  constraint symmetric L61 A62 A65
  constraint symmetric L61 A63 A67
  constraint symmetric L62 A60 A71
  constraint symmetric L62 A61 A73
  constraint symmetric L62 A62 A70
  constraint symmetric L62 A63 A72
  constraint symmetric L62 A64 A68
  constraint symmetric L62 A65 A69
  constraint symmetric L62 A66 A74
  constraint symmetric L62 A67 A75
  measures "d47" diameter of A60
  measures "d48" diameter of A61
  measures "d49" diameter of A62
  measures "d50" diameter of A63
extrude "Extrude5" cut sketch "Sketch4" against normal blind 2 contours L0 A0 L1 L68 L69 | L9 A3 L10 L66 L67 | L3 A1 L4 L70 L71 | L6 A2 L7 L72 L73 bodies 1
extrude "Extrude6" cut sketch "Sketch4" against normal blind 2 contours A60 | A61 | A62 | A63 | A64 | A65 | A66 | A67 | A68 | A69 | A70 | A71 | A72 | A73 | A74 | A75 bodies 1
sketch "Sketch5" plane through (0, 0, 2) normal (0, 0, 1) x (-1, 0, 0)
  circle A0 centre (-45, -29.2462) radius 0.75
  circle A1 centre (-23.2462, -30.2462) radius 0.75
  circle A2 centre (-23.2462, -51) radius 0.75
  circle A3 centre (-51, -51) radius 0.75
  circle A4 centre (-45, -45) radius 0.75
  circle A5 centre (-23.2462, -44) radius 0.75
  circle A6 centre (-23.2462, -23.2462) radius 0.75
  circle A7 centre (-51, -30.2462) radius 0.75
  circle A8 centre (-44, -23.2462) radius 0.75
  circle A9 centre (-29.2462, -29.2462) radius 0.75
  circle A10 centre (-30.2462, -51) radius 0.75
  circle A11 centre (-51, -44) radius 0.75
  circle A12 centre (-44, -51) radius 0.75
  circle A13 centre (-29.2462, -45) radius 0.75
  circle A14 centre (-30.2462, -23.2462) radius 0.75
  circle A15 centre (-51, -23.2462) radius 0.75
  line L0 (-53.3731, -53.3731) -> (-20.8731, -53.3731)
  line L1 (-20.8731, -53.3731) -> (-20.8731, -20.8731)
  line L2 (-20.8731, -20.8731) -> (-53.3731, -20.8731)
  line L3 (-53.3731, -20.8731) -> (-53.3731, -53.3731)
  line L4 (-43.1231, -29.1231) -> (-31.1231, -29.1231)
  line L5 (-31.1231, -29.1231) -> (-31.1231, -45.1231)
  line L6 (-31.1231, -45.1231) -> (-43.1231, -45.1231)
  line L7 (-43.1231, -45.1231) -> (-43.1231, -29.1231)
  line L8 (-43.1231, -29.1231) -> (-31.1231, -45.1231) construction
  line L9 (-31.1231, -29.1231) -> (-43.1231, -45.1231) construction
  line L10 (-34.1231, -45.1231) -> (-40.1231, -45.1231) construction
  line L11 (-31.8731, -32.1231) -> (-31.8731, -42.1231)
  arc A16 (-31.8731, -42.1231) -> (-30.3731, -42.1231) centre (-31.1231, -42.1231) ccw
  line L12 (-30.3731, -42.1231) -> (-30.3731, -32.1231)
  arc A17 (-30.3731, -32.1231) -> (-31.8731, -32.1231) centre (-31.1231, -32.1231) ccw
  line L13 (-31.1231, -32.1231) -> (-31.1231, -42.1231) construction
  line L14 (-43.8731, -32.1231) -> (-43.8731, -42.1231)
  arc A18 (-43.8731, -42.1231) -> (-42.3731, -42.1231) centre (-43.1231, -42.1231) ccw
  line L15 (-42.3731, -42.1231) -> (-42.3731, -32.1231)
  arc A19 (-42.3731, -32.1231) -> (-43.8731, -32.1231) centre (-43.1231, -32.1231) ccw
  line L16 (-43.1231, -32.1231) -> (-43.1231, -42.1231) construction
  line L17 (-33.1231, -28.3731) -> (-41.1231, -28.3731)
  arc A20 (-41.1231, -28.3731) -> (-41.1231, -29.8731) centre (-41.1231, -29.1231) ccw
  line L18 (-41.1231, -29.8731) -> (-33.1231, -29.8731)
  arc A21 (-33.1231, -29.8731) -> (-33.1231, -28.3731) centre (-33.1231, -29.1231) ccw
  line L19 (-33.1231, -29.1231) -> (-41.1231, -29.1231) construction
  line L20 (-33.1231, -44.3731) -> (-41.1231, -44.3731)
  arc A22 (-41.1231, -44.3731) -> (-41.1231, -45.8731) centre (-41.1231, -45.1231) ccw
  line L21 (-41.1231, -45.8731) -> (-33.1231, -45.8731)
  arc A23 (-33.1231, -45.8731) -> (-33.1231, -44.3731) centre (-33.1231, -45.1231) ccw
  line L22 (-33.1231, -45.1231) -> (-41.1231, -45.1231) construction
  point P0 (-37.1231, -37.1231)
  point P1 (-37.1231, -45.1231)
  point P2 (-31.1231, -37.1231)
  point P3 (-43.1231, -37.1231)
  point P4 (-37.1231, -29.1231)
  point P5 (-37.1231, -45.1231)
  dimension "d55" = 12
  dimension "d56" = 16
  dimension "d58" = 1.5
  dimension "d59" = 1.5
  dimension "d60" = 4
  dimension "d61" = 1.5
  dimension "d62" = 1.5
  constraint horizontal L4
  constraint perpendicular L4 L5
  constraint parallel L4 L6
  constraint parallel L5 L7
  constraint coincident L8 P0
  constraint coincident L9 P0
  constraint parallel L6 L10
  constraint midpoint L6 P5
  constraint midpoint L10 P5
  constraint tangent L11 A16
  constraint tangent A16 L12
  constraint parallel L11 L12
  constraint tangent L12 A17
  constraint tangent L11 A17
  constraint parallel L5 L13
  constraint midpoint L5 P2
  constraint midpoint L13 P2
  constraint tangent L14 A18
  constraint tangent A18 L15
  constraint parallel L14 L15
  constraint tangent L15 A19
  constraint tangent L14 A19
  constraint parallel L7 L16
  constraint midpoint L7 P3
  constraint midpoint L16 P3
  constraint tangent L17 A20
  constraint tangent A20 L18
  constraint parallel L17 L18
  constraint tangent L18 A21
  constraint tangent L17 A21
  constraint parallel L4 L19
  constraint midpoint L4 P4
  constraint midpoint L19 P4
  constraint tangent L20 A22
  constraint tangent A22 L21
  constraint parallel L20 L21
  constraint tangent L21 A23
  constraint tangent L20 A23
  constraint parallel L6 L22
  constraint coincident P5 P1
  constraint midpoint L22 P5
  measures "d55" distance of L5.end L6.end
  measures "d56" distance of L4.end L5.end
  measures "d58" diameter of A16
  measures "d59" diameter of A18
  measures "d60" distance of A20.centre P4
  measures "d61" diameter of A20
  measures "d62" diameter of A22
extrude "Extrude8" cut sketch "Sketch5" against normal blind 2 contours L4 L17 A20 A21 | L4 A20 L18 A21 | L7 A18 L15 A19 | L7 L14 A18 A19 | L5 A16 L12 A17 | L5 L11 A16 A17 | L6 L20 A22 A23 | L6 A22 L21 A23 bodies 1
extrude "Extrude1'" add sketch "Sketch4" along normal blind 2 separate body contours L0 A0 L1 L68 L69 | L60 A56 | L60 L68 L69 | A57 L63 | L63 L66 L67 | L9 A3 L10 L66 L67 | L3 A1 L4 L70 L71 | A58 L64 | L64 L70 L71 | L6 A2 L7 L72 L73 | A59 L65 | L65 L72 L73 makes body 2 at (63.3513, 63.3299, 2) makes body 3 at (10.9089, 63.3444, 2) makes body 4 at (63.3513, 10.9163, 2) makes body 5 at (10.9089, 10.9018, 2) in component "arms"
move_body "Move5" bodies 1 to x (1, 0, 0) y (0, 1, 0) z (0, 0, 1) at (0, 0, 3)
move_body "Move6" bodies 1 to x (1, 0, 0) y (0, 1, 0) z (0, 0, 1) at (0, 0, 1)
sketch "Sketch6" plane through (0, 0, 4) normal (0, 0, 1) x (-1, 0, 0)
  circle A0 centre (-51, -30.2462) radius 0.75
  circle A1 centre (-45, -29.2462) radius 0.75
  arc A2 (-78.0603, -1.3938) -> (-77.3603, -2.6062) centre (-77.7103, -2) ccw
  line L0 (-78.0603, -1.3938) -> (-76.5481, -0.5207)
  arc A3 (-75.8481, -1.7331) -> (-76.5481, -0.5207) centre (-76.1981, -1.1269) ccw
  line L1 (-75.8481, -1.7331) -> (-77.3603, -2.6062)
  arc A4 (-73.5462, 4) -> (-74.9462, 4) centre (-74.2462, 4) ccw
  line L2 (-73.5462, 4) -> (-73.5462, 2.2538)
  arc A5 (-74.9462, 2.2538) -> (-73.5462, 2.2538) centre (-74.2462, 2.2538) ccw
  line L3 (-74.9462, 2.2538) -> (-74.9462, 4)
  arc A6 (-71.1321, -2.6062) -> (-70.4321, -1.3938) centre (-70.7821, -2) ccw
  line L4 (-71.1321, -2.6062) -> (-72.6444, -1.7331)
  arc A7 (-71.9444, -0.5207) -> (-72.6444, -1.7331) centre (-72.2944, -1.1269) ccw
  line L5 (-71.9444, -0.5207) -> (-70.4321, -1.3938)
  arc A8 (-74.9462, -4) -> (-73.5462, -4) centre (-74.2462, -4) ccw
  line L6 (-74.9462, -4) -> (-74.9462, -2.2538)
  arc A9 (-73.5462, -2.2538) -> (-74.9462, -2.2538) centre (-74.2462, -2.2538) ccw
  line L7 (-73.5462, -2.2538) -> (-73.5462, -4)
  arc A10 (-76.5481, 0.5207) -> (-75.8481, 1.7331) centre (-76.1981, 1.1269) ccw
  line L8 (-76.5481, 0.5207) -> (-78.0603, 1.3938)
  arc A11 (-77.3603, 2.6062) -> (-78.0603, 1.3938) centre (-77.7103, 2) ccw
  line L9 (-77.3603, 2.6062) -> (-75.8481, 1.7331)
  circle A12 centre (-44, -23.2462) radius 0.75
  circle A13 centre (-51, -23.2462) radius 0.75
  arc A14 (-70.4321, 1.3938) -> (-71.1321, 2.6062) centre (-70.7821, 2) ccw
  line L10 (-70.4321, 1.3938) -> (-71.9444, 0.5207)
  arc A15 (-72.6444, 1.7331) -> (-71.9444, 0.5207) centre (-72.2944, 1.1269) ccw
  line L11 (-72.6444, 1.7331) -> (-71.1321, 2.6062)
  circle A16 centre (-74.2462, 0) radius 1
  arc A17 (-53.3731, -30.8731) -> (-43.3731, -20.8731) centre (-48.3731, -25.8731) ccw
  line L12 (-43.3731, -20.8731) -> (-64.2462, 0)
  arc A18 (-64.2462, 0) -> (-74.2462, -10) centre (-74.2462, 0) ccw
  line L13 (-74.2462, -10) -> (-53.3731, -30.8731)
  circle A19 centre (-74.2462, 0) radius 13.2902
  circle A20 centre (-74.2462, 0) radius 14
  circle A21 centre (-74.2462, -75) radius 14
  circle A22 centre (-74.2462, -75) radius 13.2902
  circle A23 centre (0, -75) radius 14
  circle A24 centre (0, -75) radius 13.2902
  circle A25 centre (0, 0) radius 14
  circle A26 centre (0, 0) radius 13.2902
  dimension "d68" = 28
  constraint concentric A16 A19
  constraint concentric A19 A20
  measures "d68" diameter of A20
sketch "Sketch7" plane through (0, 0, 6) normal (0, 0, 1) x (-1, 0, 0)
  circle A0 centre (-74.2462, 0) radius 13.2902
  circle A1 centre (-74.2462, 0) radius 14
  line L0 (-74.2462, -14) -> (-74.2462, 14)
  line L1 (-88.2462, 0) -> (-60.2462, 0)
  circle A2 centre (-74.2462, 0) radius 0.5
  line L2 (-73.7462, 0) -> (-74.7462, 0)
  line L3 (-74.7462, 0) -> (-74.7462, -13.9911)
  line L4 (-74.7462, -13.9911) -> (-73.7462, -13.9911)
  line L5 (-73.7462, -13.9911) -> (-73.7462, 0)
  line L6 (-73.7462, 0) -> (-74.7462, 0)
  line L7 (-74.7462, 0) -> (-74.7462, 13.9911)
  line L8 (-74.7462, 13.9911) -> (-73.7462, 13.9911)
  line L9 (-73.7462, 13.9911) -> (-73.7462, 0)
  line L10 (-74.2462, -0.5) -> (-88.2373, -0.5)
  line L11 (-88.2373, -0.5) -> (-88.2373, 0.5)
  line L12 (-88.2373, 0.5) -> (-74.2462, 0.5)
  line L13 (-74.2462, 0.5) -> (-74.2462, -0.5)
  line L14 (-74.2462, -0.5) -> (-60.2551, -0.5)
  line L15 (-60.2551, -0.5) -> (-60.2551, 0.5)
  line L16 (-60.2551, 0.5) -> (-74.2462, 0.5)
  line L17 (-74.2462, 0.5) -> (-74.2462, -0.5)
  dimension "d71" = 1
  dimension "d72" = 1
  dimension "d73" = 1
  dimension "d74" = 1
  constraint coincident A1 L0.start
  constraint coincident A1 L0.end
  constraint vertical L0
  constraint coincident A1 L1.start
  constraint coincident A1 L1.end
  constraint perpendicular L0 L1
  constraint concentric A0 A2
  constraint horizontal L2
  constraint vertical L3
  constraint horizontal L4
  constraint vertical L5
  constraint coincident A1 L3.end
  constraint coincident L1 L2.start
  constraint coincident A2 L2.start
  constraint horizontal L6
  constraint vertical L7
  constraint horizontal L8
  constraint vertical L9
  constraint coincident A1 L7.end
  constraint horizontal L10
  constraint vertical L11
  constraint horizontal L12
  constraint vertical L13
  constraint coincident A1 L11.end
  constraint coincident A2 L10.start
  constraint coincident L0 L10.start
  constraint horizontal L14
  constraint vertical L15
  constraint horizontal L16
  constraint vertical L17
  constraint coincident A1 L15.end
  measures "d71" diameter of A2
  measures "d72" distance of L2.start L2.end
  measures "d73" distance of L10.start L12.end
  measures "d74" distance of L10.start L12.end
extrude "Extrude2'" add sketch "Sketch6" along normal blind 1.5 from surface at 5 separate body contours L12 L13 A19 A20 | L12 L13 A19 A20 makes body 6 in component "arms"
extrude "Extrude3'" add sketch "Sketch7" along normal blind 3 from surface at 3.5 contours A0 L1 L9 L16 | A0 L1 L14 L15 | A0 L1 L5 L14 | A0 L1 L15 L16 | L0 L1 A2 L2 L6 L13 L17 | L0 L1 A2 L2 L6 L13 L17 | A2 L5 L14 | A2 L9 L16 | A0 L0 L9 L16 | A0 L0 L8 L9 | A0 L0 L4 L5 | A0 L0 L5 L14 | L0 L1 A2 L2 L6 L13 L17 | L0 L1 A2 L2 L6 L13 L17 | A0 L0 L7 L12 | A2 L7 L12 | A2 L3 L10 | A0 L0 L3 L10 | A0 L0 L7 L8 | A0 L0 L3 L4 | A0 L1 L3 L10 | A0 L1 L7 L12 | A0 L1 L11 L12 | A0 L1 L10 L11 bodies 6 in component "arms"
extrude "Extrude4" cut sketch "Sketch7" along normal blind 5.5 contours A0 L1 L9 L16 | A0 L1 L5 L14 | A0 L0 L9 L16 | A0 L0 L5 L14 | A0 L0 L7 L12 | A0 L0 L3 L10 | A0 L1 L3 L10 | A0 L1 L7 L12 bodies 6 in component "arms"
extrude "Extrude5'" cut 1 faces at (74.4129, -0.1667, 9.5) along direction (0, 0, 1) blind 2 on bodies 6 bodies 6 in component "arms"
fillet "Fillet1" radius 1 4 edges at (60.2551, 0, 12.5) (74.2462, 13.9911, 12.5) (88.2373, 0, 12.5) (74.2462, -13.9911, 12.5) on bodies 6 in component "arms"
extrude "Extrude6'" cut 1 faces at (74.3018, 4.763, 11.5) along direction (0, 0, 1) blind 0.5 on bodies 6 bodies 6 in component "arms"
fillet "Fillet2" radius 0.5 4 edges at (87.5364, 0, 12) (74.2462, 13.2902, 12) (60.956, 0, 12) (74.2462, -13.2902, 12) on bodies 6 in component "arms"
sketch "Sketch2 (2)" plane through (0, 0, 9) normal (0, 0, -1) x (1, 0, 0) in component "arms"
  circle A0 centre (74.2462, 0) radius 13.2902
  circle A1 centre (74.2462, 0) radius 14
  line L0 (87.5269, 0.5024) -> (88.2372, 0.5024)
  line L1 (87.5269, -0.5024) -> (88.2372, -0.5024)
  line L2 (60.9655, -0.5024) -> (60.2552, -0.5024)
  line L3 (60.9655, 0.5024) -> (60.2552, 0.5024)
  line L4 (74.7484, 13.2807) -> (74.7484, 13.991)
  line L5 (73.744, 13.2807) -> (73.744, 13.991)
  line L6 (73.744, -13.2807) -> (73.744, -13.991)
  line L7 (74.7484, -13.2807) -> (74.7484, -13.991)
  constraint coincident A0 L0.start
  constraint coincident A1 L0.end
  constraint horizontal L0
  constraint coincident A0 L1.start
  constraint coincident A1 L1.end
  constraint parallel L0 L1
  constraint coincident A0 L2.start
  constraint coincident A1 L2.end
  constraint parallel L1 L2
  constraint coincident A0 L3.start
  constraint coincident A1 L3.end
  constraint parallel L1 L3
  constraint coincident A0 L4.start
  constraint coincident A1 L4.end
  constraint perpendicular L3 L4
  constraint coincident A0 L5.start
  constraint coincident A1 L5.end
  constraint parallel L4 L5
  constraint coincident A0 L6.start
  constraint coincident A1 L6.end
  constraint parallel L5 L6
  constraint coincident A0 L7.start
  constraint coincident A1 L7.end
  constraint parallel L6 L7
extrude "Extrude7" add sketch "Sketch2 (2)" along normal blind 8 contours A0 A1 L0 L1 | A0 A1 L4 L5 | A0 A1 L6 L7 | A0 A1 L2 L3 bodies 6 in component "arms"
copy_body "Body->Comp1" bodies 6 removing the originals makes body 7 in component "guards"
ref_plane "WorkPlane1" through (75.0877, -13.8439, 3.9413) normal (0, 1, 0) x (0, 0, -1)
sketch "Sketch8" plane through (75.0877, -13.8439, 3.9413) normal (0, 1, 0) x (1, 0, 0)
  line L0 (-1, 3.5) -> (0, 3.5)
  line L1 (0, 3.5) -> (0, 4.5)
  line L2 (0, 4.5) -> (-1, 4.5)
  line L3 (-1, 4.5) -> (-1, 3.5)
  constraint horizontal L0
  constraint vertical L1
  constraint horizontal L2
  constraint vertical L3
extrude "Extrude1''" add sketch "Sketch8" along normal blind 28 sketch seen with x (1, 0, 0) y (0, 1, 0) z (0, 0, 1) at (-0.3392, -0.1471, 1.0587) bodies 7 in component "guards"
ref_plane "WorkPlane2" through (88.5764, 0.6495, 3.9413) normal (1, 0, 0) x (0, 0, -1)
sketch "Sketch9" plane through (88.5764, 0.6495, 3.9413) normal (1, 0, 0) x (0, 1, 0)
  line L0 (-1, -3.5) -> (0, -3.5)
  line L1 (0, -3.5) -> (0, -4.5)
  line L2 (0, -4.5) -> (-1, -4.5)
  line L3 (-1, -4.5) -> (-1, -3.5)
  constraint horizontal L0
  constraint vertical L1
  constraint horizontal L2
  constraint vertical L3
extrude "Extrude2''" add sketch "Sketch9" against normal blind 28 sketch seen with x (1, 0, 0) y (0, 1, 0) z (0, 0, 1) at (-0.3392, -0.1471, 1.0587) bodies 7 in component "guards"
sketch "Sketch10" plane through (0, 0, -0.5587) normal (0, 0, -1) x (1, 0, 0)
  line L0 (75.0877, 0.3505) -> (75.0877, 13.8439)
  line L1 (75.0877, 13.8439) -> (74.0877, 13.8439)
  line L2 (74.0877, 13.8439) -> (74.0877, 0.3505)
  line L3 (74.0877, 0.3505) -> (60.5764, 0.3505)
  line L4 (60.5764, 0.3505) -> (60.5764, -0.6495)
  line L5 (60.5764, -0.6495) -> (74.0877, -0.6495)
  line L6 (74.0877, -0.6495) -> (74.0877, -14.1561)
  line L7 (74.0877, -14.1561) -> (75.0877, -14.1561)
  line L8 (75.0877, -14.1561) -> (75.0877, -0.6495)
  line L9 (75.0877, -0.6495) -> (88.5764, -0.6495)
  line L10 (88.5764, -0.6495) -> (88.5764, 0.3505)
  line L11 (88.5764, 0.3505) -> (75.0877, 0.3505)
  line L12 (79, -5) -> (70, -5)
  line L13 (70, -5) -> (70, 5)
  line L14 (70, 5) -> (79, 5)
  line L15 (79, 5) -> (79, -5)
  line L16 (79, -5) -> (70, 5) construction
  line L17 (70, -5) -> (79, 5) construction
  point P0 (74.5, 0)
  constraint horizontal L12
  constraint perpendicular L12 L13
  constraint parallel L12 L14
  constraint parallel L13 L15
  constraint coincident L16 P0
  constraint coincident L17 P0
extrude "Extrude3''" add sketch "Sketch10" against normal blind 1 contours L0 L11 L14 L15 | L2 L3 L13 L14 | L8 L9 L12 L15 | L5 L6 L12 L13 sketch seen with x (1, 0, 0) y (0, 1, 0) z (0, 0, 1) at (-0.3392, -0.1471, 1.0587) bodies 7 in component "guards"
extrude "Extrude8'" cut sketch "Sketch2" against normal blind 5 contours L51 L53 A49 A58 | A46 L55 L60 A56 | L54 A52 A53 L59 | A47 L56 L57 A51 sketch seen with x (1, 0, 0) y (0, 1, 0) z (0, 0, 1) at (-0.3392, -0.1471, 1.0587) bodies 4 in component "arms"
extrude "Extrude9" cut sketch "Sketch2" against normal blind 20 contours A0 A50 A55 | L51 L53 A49 A58 | L52 L58 A57 A59 | A46 L55 L60 A56 | L54 A52 A53 L59 | A47 L56 L57 A51 | A48 A54 L61 L62 sketch seen with x (1, 0, 0) y (0, 1, 0) z (0, 0, 1) at (-0.0365, 0.0203, 1.0542) bodies 4 in component "arms"
extrude "Extrude4'" cut sketch "Sketch2" against normal blind 10 contours A0 A50 A55 | L51 L53 A49 A58 | L52 L58 A57 A59 | A46 L55 L60 A56 | L54 A52 A53 L59 | A47 L56 L57 A51 | A48 A54 L61 L62 sketch seen with x (1, 0, 0) y (0, 1, 0) z (0, 0, 1) at (-0.0365, 0.0203, 1.0542) bodies 7 in component "guards"
fillet "Fillet1'" radius 3 4 edges at (78.6608, -5.1471, 1) (78.6608, 4.8529, 1) (69.6608, -5.1471, 1) (69.6608, 4.8529, 1) on bodies 7 in component "guards"